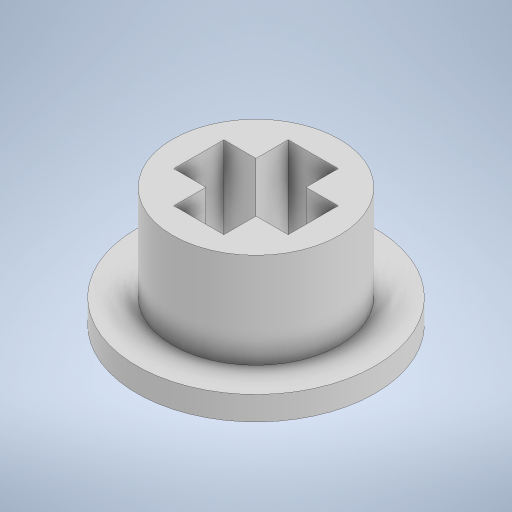
# Autodesk Inventor part: lego1
Saved by Autodesk Inventor 2023 (Build 270158000, 158)
## iProperties
Created: 2023-01-23
Part Number: lego1
Material: Ogólny
Document SubType Name: Modeling
Designer: kamil
Density: 1 g/cm^3
Appearance: Domyślna
Author: kamil
Autodesk Inventor part; units mm, degrees
ref_plane "YZ Plane" through (0, 0, 0) normal (1, 0, 0) x (0, 1, 0)
ref_plane "XZ Plane" through (0, 0, 0) normal (0, 1, 0) x (-1, 0, 0)
ref_plane "XY Plane" through (0, 0, 0) normal (0, 0, 1) x (1, 0, 0)
sketch "Szkic1" plane through (0, 0, 0) normal (0, 1, 0) x (-1, 0, 0)
  circle A0 centre (0, 0) radius 5
  circle A1 centre (0, 0) radius 3.5
  line L0 (2.4, 1.05) -> (-2.4, 1.05)
  line L1 (-2.4, 1.05) -> (-2.4, -1.05)
  line L2 (-2.4, -1.05) -> (2.4, -1.05)
  line L3 (2.4, -1.05) -> (2.4, 1.05)
  line L4 (1.05, 2.4) -> (-1.05, 2.4)
  line L5 (-1.05, 2.4) -> (-1.05, -2.4)
  line L6 (-1.05, -2.4) -> (1.05, -2.4)
  line L7 (1.05, -2.4) -> (1.05, 2.4)
  point P0 (-1.05, 0)
  point P1 (0, -1.05)
  point P2 (0, 2.4)
  point P3 (2.4, 0)
  point P4 (-1.05, 1.05)
  point P5 (1.05, 1.05)
  point P6 (1.05, -1.05)
  point P7 (-1.05, -1.05)
  dimension "d0" = 10
  dimension "d1" = 7
  dimension "d2" = 4.8
  dimension "d3" = 4.8
  dimension "d4" = 2.1
  dimension "d5" = 2.1
  constraints: 16 end point, 4 midpoint, 4 parallel, 2 centre point, 2 coincident, 2 horizontal, 2 horizontal alignment, 2 perpendicular, 2 vertical alignment
  measures "d0" diameter of A0
  measures "d1" diameter of A1
  measures "d2" distance of L4.end L5.end
  measures "d3" distance of L1.end L2.end
  measures "d4" distance of L0.end L1.end
  measures "d5" distance of L5.end L6.end
extrude "Wyciągnięcie proste1" add sketch "Szkic1" along normal blind 1 contours A0
extrude "Wyciągnięcie proste2" add sketch "Szkic1" along normal blind 5 contours A1
equation "\"d3\" = d2"
equation "\"d5\" = d4"
